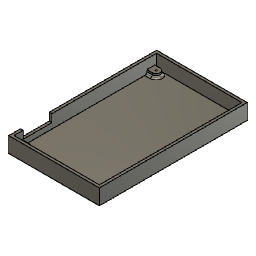
StorageChargerBase_v10 (Autodesk Fusion 360 design; units mm, degrees)
Autodesk Fusion 360 part; units mm, degrees
sketch "Sketch1" plane through (0, 0, 0) normal (0, 1, 0) x (1, 0, 0) in component "Bottom"
  arc A0 (35.8267, 60.8648) -> (34.5313, 60.8648) centre (35.179, 60.833) ccw construction
  arc A1 (35.8267, 1.6828) -> (34.5313, 1.6828) centre (35.179, 1.651) ccw construction
  line L0 (35.8267, 1.6828) -> (35.8267, 1.6192) construction
  line L1 (2.0447, 1.6828) -> (2.0447, 1.6192) construction
  line L2 (34.5313, 60.8012) -> (34.5313, 60.8648) construction
  line L3 (0, 0) -> (36.556, 0) construction
  arc A2 (34.5313, 60.8012) -> (35.8267, 60.8012) centre (35.179, 60.833) ccw construction
  line L4 (36.556, 62.408) -> (0, 62.408) construction
  arc A3 (2.0447, 1.6828) -> (0.7493, 1.6828) centre (1.397, 1.651) ccw construction
  arc A4 (0.7493, 1.6192) -> (2.0447, 1.6192) centre (1.397, 1.651) ccw construction
  line L5 (33.1175, 10.102) -> (33.1765, 10.102) construction
  line L6 (36.556, 0) -> (36.556, 62.408) construction
  line L7 (33.1765, 9.202) -> (33.1175, 9.202) construction
  line L8 (0.7493, 60.8012) -> (0.7493, 60.8648) construction
  line L9 (0.7493, 1.6192) -> (0.7493, 1.6828) construction
  arc A5 (2.0447, 60.8648) -> (0.7493, 60.8648) centre (1.397, 60.833) ccw construction
  line L10 (35.8267, 60.8648) -> (35.8267, 60.8012) construction
  line L11 (34.5313, 1.6192) -> (34.5313, 1.6828) construction
  line L12 (0, 62.408) -> (0, 0) construction
  arc A6 (0.7493, 60.8012) -> (2.0447, 60.8012) centre (1.397, 60.833) ccw construction
  arc A7 (34.5313, 1.6192) -> (35.8267, 1.6192) centre (35.179, 1.651) ccw construction
  arc A8 (33.1765, 9.202) -> (33.1765, 10.102) centre (33.147, 9.652) ccw construction
  arc A9 (33.1175, 10.102) -> (33.1175, 9.202) centre (33.147, 9.652) ccw construction
  line L13 (2.0447, 60.8648) -> (2.0447, 60.8012) construction
  circle A10 centre (1.397, 1.651) radius 0.4
  circle A11 centre (1.397, 1.651) radius 1.8
  circle A12 centre (1.397, 60.833) radius 0.4
  circle A13 centre (1.397, 60.833) radius 1.8
  circle A14 centre (35.179, 60.833) radius 0.4
  circle A15 centre (35.179, 60.833) radius 1.8
  circle A16 centre (35.179, 1.651) radius 0.4
  circle A17 centre (35.179, 1.651) radius 1.8
  line L14 (37.556, 63.408) -> (-1, 63.408)
  line L15 (-1, 63.408) -> (-1, -1)
  line L16 (-1, -1) -> (37.556, -1)
  line L17 (37.556, -1) -> (37.556, 63.408)
  line L18 (-2.2, -2.2) -> (38.756, -2.2)
  line L19 (38.756, -2.2) -> (38.756, 64.608)
  line L20 (38.756, 64.608) -> (-2.2, 64.608)
  line L21 (-2.2, 64.608) -> (-2.2, -2.2)
  line L22 (0, 3.1) -> (-5, 3.1)
  line L23 (-5, 3.1) -> (-5, 16.1)
  line L24 (-5, 16.1) -> (0, 16.1)
  line L25 (0, 16.1) -> (0, 3.1)
  line L26 (35.179, 3.451) -> (38.2, 3.451)
  line L27 (35.179, -0.149) -> (38.2, -0.149)
  line L28 (35.179, 62.633) -> (38.5, 62.633)
  line L29 (35.179, 59.033) -> (38.5, 59.033)
  line L30 (1.397, 62.633) -> (-2, 62.633)
  line L31 (1.397, 59.033) -> (-2, 59.033)
  line L32 (1.397, -0.149) -> (-2.1, -0.149)
  line L33 (1.397, 3.451) -> (-1.9, 3.451)
  point P0 (-1.397, -0.127)
  dimension "d1" = 0.8
  dimension "d2" = 1.4
  dimension "d5" = 0.8
  dimension "d6" = 1.4
  dimension "d7" = 0.8
  dimension "d8" = 1.4
  dimension "d9" = 0.8
  dimension "d10" = 1.4
  dimension "d11" = 1
  dimension "d12" = 2.2
  dimension "d21" = 3.1
  dimension "d22" = 5
  dimension "d23" = 13
  constraint concentric A3 A10
  constraint concentric A5 A12
  constraint concentric A0 A14
  constraint concentric A1 A16
  constraint horizontal L22
  constraint vertical L23
  constraint horizontal L24
  constraint vertical L25
  constraint coincident A17 L26.start
  constraint tangent A17 L26
  constraint perpendicular L17 L26
  constraint coincident A17 L27.start
  constraint tangent A17 L27
  constraint perpendicular L17 L27
  constraint coincident A15 L28.start
  constraint tangent A15 L28
  constraint perpendicular L17 L28
  constraint coincident A15 L29.start
  constraint tangent A15 L29
  constraint perpendicular L17 L29
  constraint coincident A13 L30.start
  constraint tangent A13 L30
  constraint perpendicular L15 L30
  constraint coincident A13 L31.start
  constraint tangent A13 L31
  constraint horizontal L31
  constraint coincident A11 L32.start
  constraint tangent A11 L32
  constraint perpendicular L15 L32
  constraint coincident A11 L33.start
  constraint tangent A11 L33
  constraint perpendicular L15 L33
  constraint horizontal L27
  measures "d1" diameter of A10
  measures "d5" diameter of A12
  measures "d7" diameter of A14
  measures "d9" diameter of A16
  measures "d21" distance of L3.start L22.start
  measures "d22" distance of L22.start L22.end
  measures "d23" distance of L22.start L24.end
extrude "Extrude1" add sketch "Sketch1" along normal blind 1 contours A10 | A11 | A11 A13 A15 A17 L14 L15 L16 L17 L24 L25 L26 L27 L28 L29 L30 L31 L32 L33 | A11 L15 L22 L25 L32 L33 | L15 L24 L25 L33 | L15 L22 L25 L33 | L14 L15 L16 L17 L18 L19 L20 L21 L22 L24 | L15 L21 L22 L24 | A13 L15 L30 L31 | A17 L17 L26 L27 | A13 | A17 | A15 L17 L28 L29 | A15 | A12 | A14 | A16 makes body 1 in component "Bottom"
extrude "Extrude2" add sketch "Sketch1" along normal blind 2.8 separate body contours A11 | A11 L15 L22 L25 L32 L33 | L15 L22 L25 L33 | A13 L15 L30 L31 | A17 L17 L26 L27 | A13 | A17 | A15 L17 L28 L29 | A15 makes body 2 at (2.8585, 0.9333, -59.7822) makes body 3 at (3.0377, 0.9333, -2.3913) makes body 4 at (34.2404, 1.8667, -62.3689) makes body 5 at (33.8294, 1.8667, -2.842) in component "Bottom"
extrude "Extrude3" add sketch "Sketch1" along normal blind 7 contours L14 L15 L16 L17 L18 L19 L20 L21 L22 L24 bodies 1 2 3 4 5 in component "Bottom"
extrude "Extrude4" add sketch "Sketch1" along normal blind 3.5 contours L15 L21 L22 L24 bodies 1 in component "Bottom"
fillet "Fillet1" radius 1 4 edges at (3.197, 1, -60.833) (33.379, 1, -60.833) (3.197, 1, -1.651) (33.379, 1, -1.651) on bodies 1 in component "Bottom"
component "Bottom" placed x (1, 0, 0) y (0, 1, 0) z (0, 0, 1) at (0, 0, 0)
named bodies: "StorageChargerBottom"
